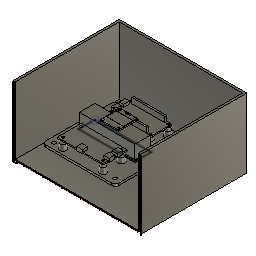
case_holder (Autodesk Fusion 360 design; units mm, degrees)
Autodesk Fusion 360 part; units mm, degrees
note: some values were not read from the file. Set by a fixed rule: which face or edge a step refers to.
sketch "Skizze1" plane through (0, 0, 0) normal (0, 0, 1) x (1, 0, 0) in component "Gehäuse"
  line L0 (0, 0) -> (175, 0)
  line L1 (175, 0) -> (175, 151)
  line L2 (175, 151) -> (0, 151)
  line L3 (0, 151) -> (0, 0)
  line L4 (3, 3) -> (172, 3)
  line L5 (172, 3) -> (172, 148)
  line L6 (172, 148) -> (3, 148)
  line L7 (3, 148) -> (3, 3)
  dimension "d1" = 175
  dimension "d2" = 151
  dimension "d3" = -3
  constraint horizontal L0
  constraint vertical L1
  constraint horizontal L2
  constraint vertical L3
  constraint coincident L0.start L3.end
  measures "d1" distance of L1.end L2.end
  measures "d2" distance of L0.start L2.end
extrude "Extrusion1" add sketch "Skizze1" along normal blind 95 makes body 1 in component "Gehäuse"
extrude "Extrusion2" add sketch "Skizze1" along normal blind 3 contours L4 L5 L6 L7 bodies 1 in component "Gehäuse"
sketch "Skizze4" plane through (0, 0, 3) normal (0, 0, 1) x (-1, 0, 0) in component "Gehäuse"
  line L0 (-3, -148) -> (-3, -3)
  line L1 (-3, -3) -> (-172, -3)
  line L2 (-172, -3) -> (-172, -148)
  line L3 (-172, -148) -> (-3, -148)
  line L4 (-3, -75.5) -> (-172, -75.5) construction
  circle A0 centre (-23.25, -75.5) radius 1.5
  line L5 (-87.5, -148) -> (-87.5, -3) construction
  circle A1 centre (-151.75, -75.5) radius 1.5
  circle A2 centre (-23.25, -75.5) radius 5
  circle A3 centre (-151.75, -75.5) radius 5
  dimension "d207" = 128.5
  dimension "d208" = 3
  dimension "d211" = 10
  constraint midpoint L0 L4.start
  constraint midpoint L2 L4.end
  constraint coincident L4 A0.centre
  constraint midpoint L3 L5.start
  constraint midpoint L1 L5.end
  constraint symmetric A0 L5 A1
  constraint concentric A0 A2
  constraint symmetric L5 A2 A3
  measures "d207" distance of A0.centre A1.centre
  measures "d208" diameter of A0
  measures "d211" diameter of A2
extrude "Extrusion3" add sketch "Skizze4" along normal blind 15 contours A2 | A3 bodies 1 in component "Gehäuse"
sketch "Skizze1 (2)" plane through (0, 0, 0) normal (0, 0, 1) x (1, 0, 0) in component "firebeetle"
  line L0 (0, 0) -> (29, 0)
  line L1 (29, 0) -> (29, 58)
  line L2 (29, 58) -> (0, 58)
  line L3 (0, 58) -> (0, 0)
  line L4 (0, 29) -> (29, 29) construction
  line L5 (14.5, 58) -> (14.5, 0) construction
  circle A0 centre (2.5, 55.5) radius 1.55
  circle A1 centre (2.5, 2.5) radius 1.55
  circle A2 centre (26.5, 55.5) radius 1.55
  circle A3 centre (26.5, 2.5) radius 1.55
  line L6 (0.55, 51.5) -> (3.05, 51.5)
  line L7 (3.05, 51.5) -> (3.05, 6.5)
  line L8 (3.05, 6.5) -> (0.55, 6.5)
  line L9 (0.55, 6.5) -> (0.55, 51.5)
  line L10 (1.8, 51.5) -> (1.8, 6.5) construction
  line L11 (0.55, 29) -> (3.05, 29) construction
  line L12 (28.45, 6.5) -> (28.45, 51.5)
  line L13 (28.45, 51.5) -> (25.95, 51.5)
  line L14 (25.95, 6.5) -> (28.45, 6.5)
  line L15 (25.95, 51.5) -> (25.95, 6.5)
  line L16 (27.2, 51.5) -> (27.2, 6.5) construction
  line L17 (28.45, 29) -> (25.95, 29) construction
  line L18 (5, 59) -> (13, 59)
  line L19 (13, 59) -> (13, 53)
  line L20 (13, 53) -> (5, 53)
  line L21 (5, 53) -> (5, 59)
  line L22 (16, 59) -> (24, 59)
  line L23 (24, 59) -> (24, 53)
  line L24 (24, 53) -> (16, 53)
  line L25 (16, 53) -> (16, 59)
  dimension "d8" = 58
  dimension "d9" = 29
  dimension "d10" = 53
  dimension "d11" = 24
  dimension "d12" = 3.1
  dimension "d13" = 25.4
  dimension "d14" = 45
  dimension "d15" = 2.5
  dimension "d20" = 8
  dimension "d21" = 8
  dimension "d22" = 6
  dimension "d23" = 6
  dimension "d24" = 1.5
  dimension "d25" = 1.5
  dimension "d26" = 1
  dimension "d27" = 1
  constraint horizontal L0
  constraint vertical L1
  constraint horizontal L2
  constraint vertical L3
  constraint coincident L0.start L3.end
  constraint midpoint L3 L4.start
  constraint midpoint L1 L4.end
  constraint midpoint L2 L5.start
  constraint midpoint L0 L5.end
  constraint symmetric L4 A0 A1
  constraint symmetric L5 A0 A2
  constraint symmetric L5 A1 A3
  constraint horizontal L6
  constraint vertical L7
  constraint horizontal L8
  constraint vertical L9
  constraint midpoint L6 L10.start
  constraint midpoint L8 L10.end
  constraint midpoint L9 L11.start
  constraint midpoint L7 L11.end
  constraint symmetric L5 L6.start L12.end
  constraint symmetric L5 L6.end L13.end
  constraint symmetric L5 L7.end L14.start
  constraint symmetric L5 L8.end L12.start
  constraint symmetric L5 L10.start L16.start
  constraint symmetric L5 L10.end L16.end
  constraint symmetric L5 L11.start L17.start
  constraint symmetric L5 L11.end L17.end
  constraint collinear L4 L11
  constraint horizontal L18
  constraint vertical L19
  constraint horizontal L20
  constraint vertical L21
  constraint horizontal L22
  constraint vertical L23
  constraint horizontal L24
  constraint vertical L25
  measures "d8" distance of L0.start L2.end
  measures "d9" distance of L1.end L2.end
  measures "d10" distance of A0.centre A1.centre
  measures "d11" distance of A1.centre A3.centre
  measures "d12" diameter of A0
  measures "d13" distance of L10 L16
  measures "d14" distance of L6.end L7.end
  measures "d15" distance of L7.end L8.end
  measures "d20" distance of L18.start L18.end
  measures "d21" distance of L22.start L22.end
  measures "d22" distance of L22.start L24.end
  measures "d23" distance of L18.end L19.end
  measures "d24" distance of L5 L19
  measures "d25" distance of L5 L25
  measures "d26" distance of L2 L22
  measures "d27" distance of L2 L18
extrude "Extrusion1'" add sketch "Skizze1 (2)" along normal blind 1.6 separate body contours L0 L1 L2 L3 L19 L20 L21 L23 L24 L25 | L2 L19 L20 L21 | L2 L23 L24 L25 makes body 2 in component "firebeetle"
extrude "Extrusion2'" add sketch "Skizze1 (2)" along normal blind 9 contours L6 L7 L8 L9 | L12 L13 L14 L15 bodies 2 in component "firebeetle"
extrude "Extrusion3'" add sketch "Skizze1 (2)" along normal blind 5 contours L2 L18 L19 L21 | L2 L19 L20 L21 | L2 L23 L24 L25 | L2 L22 L23 L25 bodies 2 in component "firebeetle"
fillet "Abrundung1" radius 2 4 edges at (29, 0, 0.8) (0, 0, 0.8) (29, 58, 0.8) (0, 58, 0.8) on bodies 2 in component "firebeetle"
sketch "Skizze1 (3)" plane through (0, 0, 0) normal (0, 0, 1) x (1, 0, 0) in component "OLED Display"
  line L0 (0, 0) -> (25, 0)
  line L1 (25, 0) -> (25, 27)
  line L2 (25, 27) -> (0, 27)
  line L3 (0, 27) -> (0, 0)
  line L4 (12.5, 27) -> (12.5, 0) construction
  line L5 (0, 13.5) -> (25, 13.5) construction
  circle A0 centre (2, 25) radius 1.4
  circle A1 centre (23, 25) radius 1.4
  circle A2 centre (2, 2) radius 1.4
  circle A3 centre (23, 2) radius 1.4
  line L6 (18, 25.5) -> (6.5174, 25.5) construction
  circle A4 centre (9.5, 25.5) radius 0.75
  circle A5 centre (11.5, 25.5) radius 0.75
  circle A6 centre (13.5, 25.5) radius 0.75
  circle A7 centre (15.5, 25.5) radius 0.75
  line L7 (0.75, 21.25) -> (24.25, 21.25)
  line L8 (24.25, 21.25) -> (24.25, 7.75)
  line L9 (24.25, 7.75) -> (0.75, 7.75)
  line L10 (0.75, 7.75) -> (0.75, 21.25)
  line L11 (12.5, 21.25) -> (12.5, 7.75) construction
  line L12 (0.75, 14.5) -> (24.25, 14.5) construction
  dimension "d32" = 25
  dimension "d33" = 27
  dimension "d34" = 2.8
  dimension "d35" = 2
  dimension "d36" = 2
  dimension "d37" = 1.5
  dimension "d38" = 1.5
  dimension "d39" = 2
  dimension "d40" = 2
  dimension "d41" = 2
  dimension "d42" = 1
  dimension "d43" = 13.5
  dimension "d44" = 23.5
  dimension "d45" = 1
  constraint horizontal L0
  constraint vertical L1
  constraint horizontal L2
  constraint vertical L3
  constraint coincident L0.start L3.end
  constraint midpoint L2 L4.start
  constraint midpoint L0 L4.end
  constraint midpoint L3 L5.start
  constraint midpoint L1 L5.end
  constraint symmetric L4 A0 A1
  constraint symmetric L5 A0 A2
  constraint symmetric L5 A1 A3
  constraint perpendicular L4 L6
  constraint coincident L6 A4.centre
  constraint coincident L6 A5.centre
  constraint coincident L6 A6.centre
  constraint coincident L6 A7.centre
  constraint equal A4 A5
  constraint equal A4 A6
  constraint equal A4 A7
  constraint horizontal L7
  constraint vertical L8
  constraint horizontal L9
  constraint vertical L10
  constraint midpoint L7 L11.start
  constraint midpoint L9 L11.end
  constraint midpoint L10 L12.start
  constraint midpoint L8 L12.end
  constraint collinear L4 L11
  measures "d32" distance of L1.end L2.end
  measures "d33" distance of L0.end L1.end
  measures "d34" diameter of A0
  measures "d35" distance of L2 A0.centre
  measures "d36" distance of L3 A0.centre
  measures "d37" distance of L2 L6
  measures "d38" diameter of A4
  measures "d39" distance of A4.centre A5.centre
  measures "d40" distance of A5.centre A6.centre
  measures "d41" distance of A6.centre A7.centre
  measures "d42" distance of L4 A6.centre
  measures "d43" distance of L7.end L8.end
  measures "d44" distance of L8.end L9.end
  measures "d45" distance of L5 L12
extrude "Extrusion1''" add sketch "Skizze1 (3)" along normal blind 1.6 separate body makes body 3 in component "OLED Display"
extrude "Extrusion2''" add sketch "Skizze1 (3)" along normal blind 2 contours L7 L8 L9 L10 bodies 3 in component "OLED Display"
extrude "Extrusion3''" add sketch "Skizze1 (3)" along normal blind 3 contours A4 | A5 | A6 | A7 bodies 3 in component "OLED Display"
sketch "Skizze1 (4)" plane through (0, 0, 0) normal (0, 0, 1) x (1, 0, 0) in component "Solar Manager 5v"
  line L0 (0, 0) -> (63, 0)
  line L1 (63, 0) -> (63, 33)
  line L2 (63, 33) -> (0, 33)
  line L3 (0, 33) -> (0, 0)
  line L4 (31.5, 33) -> (31.5, 0) construction
  line L5 (0, 16.5) -> (63, 16.5) construction
  circle A0 centre (4, 29) radius 1.6
  circle A1 centre (59, 29) radius 1.6
  circle A2 centre (4, 4) radius 1.6
  circle A3 centre (59, 4) radius 1.6
  line L6 (-1, 26) -> (6, 26)
  line L7 (6, 26) -> (6, 18)
  line L8 (6, 18) -> (-1, 18)
  line L9 (-1, 18) -> (-1, 26)
  line L10 (-1, 15) -> (6, 15)
  line L11 (6, 15) -> (6, 7)
  line L12 (6, 7) -> (-1, 7)
  line L13 (-1, 7) -> (-1, 15)
  line L14 (27.5, 34) -> (35.5, 34)
  line L15 (35.5, 34) -> (35.5, 27)
  line L16 (35.5, 27) -> (27.5, 27)
  line L17 (27.5, 27) -> (27.5, 34)
  dimension "d52" = 63
  dimension "d53" = 33
  dimension "d54" = 55
  dimension "d55" = 25
  dimension "d56" = 3.2
  dimension "d57" = 8
  dimension "d58" = 8
  dimension "d59" = 8
  dimension "d60" = 7
  dimension "d61" = 7
  dimension "d62" = 7
  dimension "d63" = 1
  dimension "d64" = 4
  dimension "d65" = 1
  dimension "d66" = 1
  dimension "d67" = 1.5
  dimension "d68" = 1.5
  constraint horizontal L0
  constraint vertical L1
  constraint horizontal L2
  constraint vertical L3
  constraint coincident L0.start L3.end
  constraint midpoint L2 L4.start
  constraint midpoint L0 L4.end
  constraint midpoint L3 L5.start
  constraint midpoint L1 L5.end
  constraint symmetric L4 A0 A1
  constraint symmetric L5 A0 A2
  constraint symmetric L5 A1 A3
  constraint horizontal L6
  constraint vertical L7
  constraint horizontal L8
  constraint vertical L9
  constraint horizontal L10
  constraint vertical L11
  constraint horizontal L12
  constraint vertical L13
  constraint horizontal L14
  constraint vertical L15
  constraint horizontal L16
  constraint vertical L17
  measures "d52" distance of L1.end L2.end
  measures "d53" distance of L0.start L2.end
  measures "d54" distance of A0.centre A1.centre
  measures "d55" distance of A0.centre A2.centre
  measures "d56" diameter of A0
  measures "d57" distance of L14.start L14.end
  measures "d58" distance of L6.start L8.end
  measures "d59" distance of L10.start L12.end
  measures "d60" distance of L10.start L10.end
  measures "d61" distance of L7.end L8.end
  measures "d62" distance of L14.end L15.end
  measures "d63" distance of L2 L14
  measures "d64" distance of L4 L17
  measures "d65" distance of L3 L9
  measures "d66" distance of L3 L13
  measures "d67" distance of L5 L8
  measures "d68" distance of L5 L10
extrude "Extrusion1'''" add sketch "Skizze1 (4)" along normal blind 1.6 separate body contours L0 L1 L2 L3 L6 L7 L8 L10 L11 L12 L15 L16 L17 makes body 4 in component "Solar Manager 5v"
extrude "Extrusion2'''" add sketch "Skizze1 (4)" along normal blind 5 contours L3 L10 L12 L13 | L3 L10 L11 L12 | L2 L15 L16 L17 | L2 L14 L15 L17 | L3 L6 L8 L9 | L3 L6 L7 L8 bodies 4 in component "Solar Manager 5v"
sketch "Skizze1 (5)" plane through (0, 0, 0) normal (0, 0, 1) x (1, 0, 0) in component "Relais"
  line L0 (0, 0) -> (40, 0)
  line L1 (40, 0) -> (40, 40)
  line L2 (40, 40) -> (0, 40)
  line L3 (0, 40) -> (0, 0)
  line L4 (4.5, 10.5) -> (35.5, 10.5)
  line L5 (35.5, 10.5) -> (35.5, 2.5)
  line L6 (35.5, 2.5) -> (4.5, 2.5)
  line L7 (4.5, 2.5) -> (4.5, 10.5)
  line L8 (20, 10.5) -> (20, 2.5)
  line L9 (20, 40) -> (20, 0) construction
  line L10 (15, 31.5) -> (25, 31.5)
  line L11 (25, 31.5) -> (25, 11.5)
  line L12 (25, 11.5) -> (15, 11.5)
  line L13 (15, 11.5) -> (15, 31.5)
  line L14 (20, 31.5) -> (20, 11.5) construction
  line L15 (15, 39) -> (25, 39)
  line L16 (25, 39) -> (25, 34)
  line L17 (25, 34) -> (15, 34)
  line L18 (15, 34) -> (15, 39)
  line L19 (20, 39) -> (20, 34) construction
  circle A0 centre (10, 40) radius 1.5
  circle A1 centre (40, 30) radius 1.5
  circle A2 centre (0, 10) radius 1.5
  circle A3 centre (30, 0) radius 1.5
  dimension "d73" = 40
  dimension "d74" = 40
  dimension "d75" = 31
  dimension "d76" = 8
  dimension "d77" = 2.5
  dimension "d78" = 20
  dimension "d79" = 10
  dimension "d80" = 1
  dimension "d81" = 10
  dimension "d82" = 5
  dimension "d83" = 1
  dimension "d84" = 3
  dimension "d85" = 10
  dimension "d86" = 3
  dimension "d87" = 3
  dimension "d88" = 3
  dimension "d89" = 10
  dimension "d90" = 10
  dimension "d91" = 10
  constraint horizontal L0
  constraint vertical L1
  constraint horizontal L2
  constraint vertical L3
  constraint coincident L0.start L3.end
  constraint horizontal L4
  constraint vertical L5
  constraint horizontal L6
  constraint vertical L7
  constraint midpoint L4 L8.start
  constraint midpoint L6 L8.end
  constraint midpoint L2 L9.start
  constraint midpoint L0 L9.end
  constraint collinear L8 L9
  constraint horizontal L10
  constraint vertical L11
  constraint horizontal L12
  constraint vertical L13
  constraint midpoint L10 L14.start
  constraint midpoint L12 L14.end
  constraint collinear L9 L14
  constraint horizontal L15
  constraint vertical L16
  constraint horizontal L17
  constraint vertical L18
  constraint midpoint L15 L19.start
  constraint midpoint L17 L19.end
  constraint collinear L9 L19
  constraint coincident L2 A0.centre
  constraint coincident L1 A1.centre
  constraint coincident L3 A2.centre
  constraint coincident L0 A3.centre
  measures "d73" distance of L1.end L2.end
  measures "d74" distance of L0.end L1.end
  measures "d75" distance of L4.start L4.end
  measures "d76" distance of L4.end L5.end
  measures "d77" distance of L0 L6
  measures "d78" distance of L10.end L11.end
  measures "d79" distance of L10.start L10.end
  measures "d80" distance of L4 L12
  measures "d81" distance of L15.start L15.end
  measures "d82" distance of L15.end L16.end
  measures "d83" distance of L2 L15
  measures "d84" diameter of A0
  measures "d85" distance of L3 A0.centre
  measures "d86" diameter of A1
  measures "d87" diameter of A2
  measures "d88" diameter of A3
  measures "d89" distance of L1 A3.centre
  measures "d90" distance of L2 A1.centre
  measures "d91" distance of L0 A2.centre
extrude "Extrusion1''''" add sketch "Skizze1 (5)" along normal blind 1.6 separate body contours L0 L1 L2 L3 A0 A1 A2 A3 makes body 5 in component "Relais"
extrude "Extrusion2''''" add sketch "Skizze1 (5)" along normal blind 5 contours L15 L16 L17 L18 bodies 5 in component "Relais"
extrude "Extrusion3'''" add sketch "Skizze1 (5)" along normal blind 10 contours L10 L11 L12 L13 bodies 5 in component "Relais"
extrude "Extrusion4" add sketch "Skizze1 (5)" along normal blind 9 contours L4 L6 L7 L8 | L4 L5 L6 L8 bodies 5 in component "Relais"
extrude "Extrusion4'" add sketch "Skizze1 (2)" against normal blind 10 contours L6 L7 L8 L9 | L12 L13 L14 L15 bodies 2 in component "firebeetle"
sketch "Skizze1 (6)" plane through (0, 0, 0) normal (0, 0, 1) x (1, 0, 0) in component "18650 Holder"
  line L0 (0, 0) -> (21.2, 0)
  line L1 (21.2, 0) -> (21.2, 76)
  line L2 (21.2, 76) -> (0, 76)
  line L3 (0, 76) -> (0, 0)
  line L4 (-1, -1) -> (22.2, -1)
  line L5 (22.2, -1) -> (22.2, 77)
  line L6 (22.2, 77) -> (-1, 77)
  line L7 (-1, 77) -> (-1, -1)
  dimension "d106" = 21.2
  dimension "d107" = 76
  dimension "d108" = 1
  constraint horizontal L0
  constraint vertical L1
  constraint horizontal L2
  constraint vertical L3
  constraint coincident L0.start L3.end
  measures "d106" distance of L1.end L2.end
  measures "d107" distance of L0.end L1.end
extrude "Extrusion1'''''" add sketch "Skizze1 (6)" along normal blind 20 separate body contours L0 L1 L2 L3 makes body 6 in component "18650 Holder"
extrude "Extrusion2'''''" add sketch "Skizze1 (6)" along normal blind 1 contours L0 L1 L2 L3 | L4 L5 L6 L7 bodies 6 in component "18650 Holder"
sketch "Skizze1 (7)" plane through (0, 0, 18) normal (0, 0, 1) x (-1, 0, 0) in component "Halterung"
  line L0 (-3, -148) -> (-3, -3)
  line L1 (-3, -3) -> (-172, -3)
  line L2 (-172, -3) -> (-172, -148)
  line L3 (-172, -148) -> (-3, -148)
  line L4 (-20, -125.5) -> (-155, -125.5)
  line L5 (-155, -125.5) -> (-155, -25.5)
  line L6 (-155, -25.5) -> (-20, -25.5)
  line L7 (-20, -25.5) -> (-20, -125.5)
  line L8 (-20, -75.5) -> (-155, -75.5) construction
  line L9 (-3, -75.5) -> (-172, -75.5) construction
  line L10 (-87.5, -148) -> (-87.5, -3) construction
  line L11 (-87.5, -125.5) -> (-87.5, -25.5) construction
  circle A0 centre (-151.75, -75.5) radius 1.5 construction
  circle A1 centre (-151.75, -75.5) radius 1.75
  circle A2 centre (-23.25, -75.5) radius 1.5
  circle A3 centre (-151.75, -75.5) radius 1.5
  circle A4 centre (-23.25, -75.5) radius 1.75
  dimension "d173" = 135
  dimension "d174" = 100
  dimension "d213" = 3.5
  dimension "d218" = 3.5
  constraint horizontal L4
  constraint vertical L5
  constraint horizontal L6
  constraint vertical L7
  constraint midpoint L5 L8.end
  constraint midpoint L0 L9.start
  constraint midpoint L2 L9.end
  constraint midpoint L3 L10.start
  constraint midpoint L1 L10.end
  constraint midpoint L4 L11.start
  constraint midpoint L6 L11.end
  constraint collinear L10 L11
  constraint collinear L8 L9
  constraint concentric A0 A1
  constraint concentric A2 A4
  measures "d173" distance of L4.start L4.end
  measures "d174" distance of L4.start L6.end
  measures "d213" diameter of A1
  measures "d218" diameter of A4
extrude "Extrusion1''''''" add sketch "Skizze1 (7)" along normal blind 3 separate body contours L4 L5 L6 L7 makes body 7 in component "Halterung"
sketch "Skizze3" plane through (0, 0, 21) normal (0, 0, 1) x (-1, 0, 0) in component "Halterung"
  line L0 (-20, -25.5) -> (-155, -25.5)
  line L1 (-155, -25.5) -> (-155, -125.5)
  line L2 (-155, -125.5) -> (-20, -125.5)
  line L3 (-20, -125.5) -> (-20, -25.5)
  line L4 (-100, -125.5) -> (-100, -25.5)
  circle A0 centre (-151.75, -75.5) radius 1.75
  circle A1 centre (-23.25, -75.5) radius 1.75
  dimension "d115" = 80
  constraint coincident L2 L4.start
  constraint coincident L0 L4.end
  constraint perpendicular L0 L4
  measures "d115" distance of L3 L4
sketch "Skizze4 (2)" plane through (0, 0, 21) normal (0, 0, 1) x (-1, 0, 0) in component "Halterung"
  line L0 (-20, -25.5) -> (-155, -25.5)
  line L1 (-155, -25.5) -> (-155, -125.5)
  line L2 (-155, -125.5) -> (-20, -125.5)
  line L3 (-20, -125.5) -> (-20, -25.5)
  circle A0 centre (-97.5, -120.5) radius 1.55 construction
  circle A1 centre (-44.5, -120.5) radius 1.55 construction
  circle A2 centre (-97.5, -96.5) radius 1.55 construction
  circle A3 centre (-44.5, -96.5) radius 1.55 construction
  circle A4 centre (-41, -58) radius 1.6 construction
  circle A5 centre (-96, -58) radius 1.6 construction
  circle A6 centre (-41, -33) radius 1.6 construction
  circle A7 centre (-96, -33) radius 1.6 construction
  line L4 (-152, -81.75) -> (-152, -110.25) construction
  arc A8 (-152, -113.25) -> (-152, -110.25) centre (-152, -111.75) ccw construction
  line L5 (-152, -113.25) -> (-152, -121.75) construction
  line L6 (-152, -121.75) -> (-123.5, -121.75) construction
  arc A9 (-120.5, -121.75) -> (-123.5, -121.75) centre (-122, -121.75) ccw construction
  line L7 (-120.5, -121.75) -> (-112, -121.75) construction
  line L8 (-112, -121.75) -> (-112, -93.25) construction
  arc A10 (-112, -90.25) -> (-112, -93.25) centre (-112, -91.75) ccw construction
  line L9 (-112, -90.25) -> (-112, -81.75) construction
  line L10 (-112, -81.75) -> (-140.5, -81.75) construction
  arc A11 (-143.5, -81.75) -> (-140.5, -81.75) centre (-142, -81.75) ccw construction
  line L11 (-143.5, -81.75) -> (-152, -81.75) construction
  circle A12 centre (-67, -78) radius 1.5
  circle A13 centre (-97.5, -96.5) radius 1.55
  circle A14 centre (-97.5, -120.5) radius 1.55
  circle A15 centre (-44.5, -120.5) radius 1.55
  circle A16 centre (-44.5, -96.5) radius 1.55
  circle A17 centre (-112, -91.75) radius 1.55
  circle A18 centre (-122, -121.75) radius 1.55
  circle A19 centre (-152, -111.75) radius 1.55
  circle A20 centre (-142, -81.75) radius 1.55
  circle A21 centre (-96, -58) radius 1.55
  circle A22 centre (-41, -58) radius 1.55
  circle A23 centre (-96, -33) radius 1.55
  circle A24 centre (-41, -33) radius 1.55
  circle A25 centre (-44.5, -120.5) radius 3.5
  circle A26 centre (-97.5, -120.5) radius 3.5
  circle A27 centre (-97.5, -96.5) radius 3.5
  circle A28 centre (-44.5, -96.5) radius 3.5
  circle A29 centre (-122, -121.75) radius 3.5
  circle A30 centre (-152, -111.75) radius 2.75
  circle A31 centre (-112, -91.75) radius 3.5
  circle A32 centre (-142, -81.75) radius 3.5
  circle A33 centre (-96, -58) radius 3.5
  circle A34 centre (-96, -33) radius 3.5
  circle A35 centre (-41, -33) radius 3.5
  circle A36 centre (-41, -58) radius 3.5
  line L12 (-105, -88.6) -> (-105, -67.4) construction
  line L13 (-105, -67.4) -> (-29, -67.4) construction
  line L14 (-29, -67.4) -> (-29, -88.6) construction
  line L15 (-29, -88.6) -> (-105, -88.6) construction
  line L16 (-29, -78) -> (-105, -78) construction
  line L17 (-67, -88.6) -> (-67, -67.4) construction
  line L18 (-105.3, -88.9) -> (-105.3, -67.1)
  line L19 (-105.3, -67.1) -> (-28.7, -67.1)
  line L20 (-28.7, -67.1) -> (-28.7, -88.9)
  line L21 (-28.7, -88.9) -> (-105.3, -88.9)
  line L22 (-106.8, -90.4) -> (-106.8, -65.6)
  line L23 (-106.8, -65.6) -> (-27.2, -65.6)
  line L24 (-27.2, -65.6) -> (-27.2, -90.4)
  line L25 (-27.2, -90.4) -> (-106.8, -90.4)
  circle A37 centre (-151.75, -75.5) radius 1.75
  circle A38 centre (-23.25, -75.5) radius 1.75
  dimension "d132" = 3
  dimension "d133" = 3.1
  dimension "d134" = 3.1
  dimension "d135" = 3.1
  dimension "d136" = 3.1
  dimension "d137" = 3.1
  dimension "d138" = 3.1
  dimension "d139" = 3.1
  dimension "d140" = 3.1
  dimension "d141" = 3.1
  dimension "d142" = 3.1
  dimension "d143" = 3.1
  dimension "d144" = 3.1
  dimension "d145" = 7
  dimension "d146" = 7
  dimension "d147" = 7
  dimension "d148" = 7
  dimension "d149" = 7
  dimension "d150" = 5.5
  dimension "d151" = 7
  dimension "d152" = 7
  dimension "d153" = 7
  dimension "d154" = 7
  dimension "d155" = 7
  dimension "d156" = 7
  dimension "d202" = -0.3
  dimension "d203" = -1.8
  constraint concentric A2 A13
  constraint concentric A0 A14
  constraint concentric A1 A15
  constraint concentric A3 A16
  constraint concentric A10 A17
  constraint concentric A9 A18
  constraint concentric A8 A19
  constraint concentric A11 A20
  constraint concentric A5 A21
  constraint concentric A4 A22
  constraint concentric A7 A23
  constraint concentric A6 A24
  constraint concentric A15 A25
  constraint concentric A14 A26
  constraint concentric A2 A27
  constraint concentric A3 A28
  constraint concentric A18 A29
  constraint concentric A8 A30
  constraint concentric A17 A31
  constraint concentric A20 A32
  constraint concentric A5 A33
  constraint concentric A23 A34
  constraint concentric A6 A35
  constraint concentric A4 A36
  constraint midpoint L14 L16.start
  constraint midpoint L12 L16.end
  constraint midpoint L15 L17.start
  constraint midpoint L13 L17.end
  constraint coincident A12.centre L17
  constraint coincident A12.centre L16
  measures "d132" diameter of A12
  measures "d133" diameter of A15
  measures "d134" diameter of A14
  measures "d135" diameter of A13
  measures "d136" diameter of A16
  measures "d137" diameter of A18
  measures "d138" diameter of A19
  measures "d139" diameter of A17
  measures "d140" diameter of A20
  measures "d141" diameter of A21
  measures "d142" diameter of A23
  measures "d143" diameter of A22
  measures "d144" diameter of A24
  measures "d145" diameter of A25
  measures "d146" diameter of A26
  measures "d147" diameter of A27
  measures "d148" diameter of A28
  measures "d149" diameter of A29
  measures "d150" diameter of A30
  measures "d151" diameter of A32
  measures "d152" diameter of A31
  measures "d153" diameter of A33
  measures "d154" diameter of A36
  measures "d155" diameter of A34
  measures "d156" diameter of A35
extrude "Extrusion2''''''" add sketch "Skizze4 (2)" along normal blind 12 contours A25 | A26 | A27 | A28 bodies 7 in component "Halterung"
extrude "Extrusion3''''" add sketch "Skizze4 (2)" along normal blind 12 contours A33 | A34 | A35 | A36 bodies 7 in component "Halterung"
extrude "Extrusion4''" add sketch "Skizze4 (2)" along normal blind 3 contours A29 | A30 | A31 | A32 bodies 7 in component "Halterung"
chamfer "Fase1" distance 1 distance2 7 8 edges at (44.2631, 56.7343, 21) (44.2631, 31.7343, 21) (99.2631, 31.7343, 21) (99.2631, 56.7343, 21) (100.7631, 95.2343, 21) (100.7631, 119.2343, 21) (47.7631, 95.2343, 21) (47.7631, 119.2343, 21) measured on face at (131.6886, 53.6534, 21) measured on face at (131.6886, 53.6534, 21) measured on face at (131.6886, 53.6534, 21) measured on face at (131.6886, 53.6534, 21) measured on face at (131.6886, 53.6534, 21) measured on face at (131.6886, 53.6534, 21) measured on face at (131.6886, 53.6534, 21) measured on face at (131.6886, 53.6534, 21) on bodies 7 in component "Halterung"
chamfer "Fase1" distance 1 distance2 2 4 edges at (115.2631, 90.4843, 21) (145.2631, 80.4843, 21) (154.5639, 110.7556, 21) (125.2631, 120.4843, 21) measured on face at (131.6886, 53.6534, 21) measured on face at (131.6886, 53.6534, 21) measured on face at (131.6886, 53.6534, 21) measured on face at (131.6886, 53.6534, 21) on bodies 7 in component "Halterung"
extrude "Extrusion5" add sketch "Skizze4 (2)" along normal blind 2 contours L22 L23 L24 L25 bodies 7 in component "Halterung"
extrude "Extrusion6" cut sketch "Skizze4 (2)" against normal up to surface (3 mm away) contours A12 bodies 7 in component "Halterung"
sketch "Skizze5" plane through (0, 0, 21) normal (0, 0, 1) x (-1, 0, 0) in component "Halterung"
  circle A0 centre (-142, -81.75) radius 4.5
  circle A1 centre (-41, -33) radius 4.5
  circle A2 centre (-96, -33) radius 4.5
  circle A3 centre (-112, -91.75) radius 4.5
  line L0 (-20, -125.5) -> (-20, -25.5)
  line L1 (-20, -25.5) -> (-155, -25.5)
  line L2 (-155, -25.5) -> (-155, -109.5)
  line L3 (-119.5125, -125.5) -> (-20, -125.5)
  line L4 (-155, -70.5) -> (-130, -70.5)
  line L5 (-120, -60.5) -> (-120, -25.5)
  arc A4 (-130, -70.5) -> (-120, -60.5) centre (-130, -60.5) ccw
  line L6 (-20, -25.5) -> (-155, -25.5)
  line L7 (-155, -25.5) -> (-155, -125.5)
  circle A5 centre (-97.5, -120.5) radius 4.5
  circle A6 centre (-44.5, -120.5) radius 4.5
  circle A7 centre (-44.5, -96.5) radius 4.5
  circle A8 centre (-97.5, -96.5) radius 4.5
  circle A9 centre (-96, -58) radius 4.5
  circle A10 centre (-41, -58) radius 4.5
  circle A11 centre (-28, -33.5) radius 2.25
  circle A12 centre (-28, -117.5) radius 2.25
  circle A13 centre (-112, -33.5) radius 2.25
  line L8 (-27.2, -90.4) -> (-106.8, -90.4)
  line L9 (-106.8, -90.4) -> (-106.8, -65.6)
  line L10 (-106.8, -65.6) -> (-27.2, -65.6)
  line L11 (-27.2, -65.6) -> (-27.2, -90.4)
  circle A14 centre (-106, -115.5) radius 2.25
  line L12 (-100, -96) -> (-100, -121)
  circle A15 centre (-151.75, -75.5) radius 1.75
  arc A16 (-119.5125, -125.5) -> (-124.4875, -125.5) centre (-122, -121.75) ccw
  arc A17 (-155, -114) -> (-155, -109.5) centre (-152, -111.75) ccw
  line L13 (-155, -114) -> (-155, -125.5)
  line L14 (-155, -125.5) -> (-124.4875, -125.5)
  circle A18 centre (-23.25, -75.5) radius 1.75
  dimension "d175" = 10
  dimension "d176" = 45
  dimension "d177" = 35
  dimension "d183" = 8
  dimension "d184" = 4.5
  dimension "d186" = 4.5
  dimension "d187" = 4.5
  dimension "d188" = 8
  dimension "d189" = 8
  dimension "d192" = 8
  dimension "d204" = 4.5
  dimension "d205" = 10
  dimension "d206" = 6
  constraint coincident L2 L4.start
  constraint perpendicular L2 L4
  constraint coincident L1 L5.end
  constraint perpendicular L1 L5
  constraint tangent L4 A4
  constraint tangent L5 A4
  constraint horizontal A11.centre A13.centre
  constraint vertical A11.centre A12.centre
  measures "d175" radius of A4
  measures "d176" distance of L4 L6
  measures "d177" distance of L5 L7
  measures "d183" distance of L1 A13.centre
  measures "d184" diameter of A12
  measures "d186" diameter of A13
  measures "d187" diameter of A11
  measures "d188" distance of L0 A11.centre
  measures "d189" distance of L3 A12.centre
  measures "d192" distance of L5 A13.centre
  measures "d204" diameter of A14
  measures "d205" distance of L3 A14.centre
  measures "d206" distance of A14.centre L12
extrude "Extrusion7" cut sketch "Skizze5" against normal up to surface (3 mm away) contours L1 L2 L4 L5 A4 L6 L7 bodies 7 in component "Halterung"
fillet "Abrundung1'" radius 5 5 edges at (120, 25.5, 19.5) (155, 70.5, 19.5) (155, 125.5, 19.5) (20, 125.5, 19.5) (20, 25.5, 19.5) on bodies 7 in component "Halterung"
extrude "Extrusion8" cut sketch "Skizze5" against normal up to surface (3 mm away) contours A11 | A12 | A13 | A14 bodies 7 in component "Halterung"
extrude "Extrusion9" cut 12 faces at (142.3221, 81.9999, 21) (111.5345, 91.9742, 21) (152.3221, 111.9999, 21) (121.5345, 121.9742, 21) (97.0345, 96.7242, 21) (97.0345, 120.7242, 21) (44.9269, 120.791, 21) (44.9269, 96.791, 21) (40.5502, 58.4433, 21) (96.3787, 58.5054, 21) (40.4833, 33.8079, 21) (95.5345, 32.7758, 21) along direction (0, 0, 1) up to surface end surface through (0, 0, 18) normal (0, 0, -1) offset 0 on bodies 7 bodies 7 in component "Halterung"
thread "Gewinde1" "ISO Metric profile 3.0 M3x0.5 6H" major diameter 3.086 minor diameter 2.529 pitch 0.5 angle 60 resizes the face on face at (42.9979, 120.1175, 19) on face at (42.9979, 120.1175, 29) on face at (42.9979, 96.1175, 19) on face at (42.9979, 96.1175, 29) on face at (95.9979, 120.1175, 19) on face at (95.9979, 120.1175, 29) on face at (95.9979, 96.1175, 19) on face at (95.9979, 96.1175, 29) on face at (120.4979, 121.3675, 19) on face at (120.4979, 121.3675, 23) on face at (110.4979, 91.3675, 19) on face at (110.4979, 91.3675, 23) on face at (142.7071, 83.1293, 20) on face at (142.7071, 83.1293, 23) on face at (152.7071, 113.1293, 20) on face at (152.7071, 113.1293, 23) on face at (97.0256, 59.1622, 19) on face at (97.0256, 59.1622, 29) on face at (65.8043, 77.0943, 19) on face at (39.7644, 57.0641, 19) on face at (39.7644, 57.0641, 29) on face at (39.7644, 32.0641, 19) on face at (39.7644, 32.0641, 29) on face at (97.0256, 34.1622, 19) on face at (97.0256, 34.1622, 29) on bodies 7 in component "Halterung"
component "Gehäuse" placed x (1, 0, 0) y (0, 1, 0) z (0, 0, 1) at (0, 0, 0)
component "firebeetle" placed x (0, 1, 0) y (-1, 0, 0) z (0, 0, 1) at (100, 94, 33)
component "OLED Display" placed x (1, 0, 0) y (0, 1, 0) z (0, 0, 1) at (54.5, 70.3, 42)
component "Solar Manager 5v" placed x (-1, 0, 0) y (0, -1, 0) z (0, 0, 1) at (100, 62, 33)
component "Relais" placed x (1, 0, 0) y (0, 1, 0) z (0, 0, 1) at (112, 81.75, 24)
component "18650 Holder" placed x (0, -1, 0) y (1, 0, 0) z (0, 0, 1) at (29, 88.6, 21)
component "Halterung" placed x (1, 0, 0) y (0, 1, 0) z (0, 0, 1) at (0, 0, 0)
equation "d118 = 12 mm + 1.6 mm"
equation "d126 = 12 mm + 1.6 mm"
equation "d130 = 3 mm + 1.6 mm"
equation "d134 = d133"
equation "d135 = d133"
equation "d136 = d133"
equation "d137 = d133"
equation "d138 = d133"
equation "d139 = d133"
equation "d140 = d133"
equation "d141 = d133"
equation "d142 = d133"
equation "d143 = d133"
equation "d144 = d133"
equation "d146 = d145"
equation "d147 = d145"
equation "d148 = d145"
equation "d149 = d145"
equation "d150 = d145 - 1.5 mm"
equation "d151 = d145"
equation "d152 = d145"
equation "d153 = d145"
equation "d154 = d145"
equation "d155 = d145"
equation "d156 = d145"
equation "d186 = d184"
equation "d187 = d184"
equation "d204 = d184"
named bodies: "Passage Halter"
